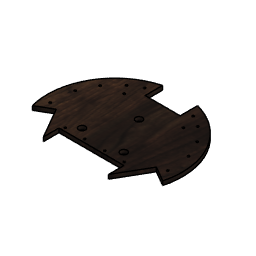
full_model (Autodesk Fusion 360 archive; units mm, degrees)
design "top"
Autodesk Fusion 360 part; units mm, degrees
sketch "Sketch1" plane through (0, 0, 0) normal (0, 0, 1) x (1, 0, 0)
  circle A0 centre (36, 80) radius 1.5
  line L0 (70.6242, -70.7971) -> (48.2374, -57.8721)
  circle A1 centre (87.282, -8.8231) radius 1.5
  circle A2 centre (51.282, -71.1769) radius 1.5
  circle A3 centre (-52.8772, 70) radius 1.5
  line L1 (0, 140) -> (0, -110) construction
  circle A4 centre (-36, 80) radius 1.5
  circle A5 centre (72.0833, 50) radius 1.5
  line L2 (-26, 96.5609) -> (26, 96.5609)
  circle A6 centre (52.8772, 70) radius 1.5
  line L3 (150, 0) -> (-170, 0) construction
  line L4 (-48.2374, -57.8721) -> (-70.6242, -70.7971)
  line L5 (26, 96.5609) -> (26, 70.7109)
  circle A7 centre (-51.282, -71.1769) radius 1.5
  circle A8 centre (-87.282, -8.8231) radius 1.5
  line L6 (-96.6242, -25.7638) -> (-74.2374, -12.8388)
  line L7 (48.2374, -57.8721) -> (74.2374, -12.8388)
  circle A9 centre (0, 0) radius 87.7268 construction
  line L8 (96.6242, -25.7638) -> (70.6242, -70.7971)
  line L9 (-74.2374, -12.8388) -> (-48.2374, -57.8721)
  line L10 (74.2374, -12.8388) -> (96.6242, -25.7638)
  circle A10 centre (84.0892, 25) radius 1.5
  circle A11 centre (0, 0) radius 100
  line L11 (-70.6242, -70.7971) -> (-96.6242, -25.7638)
  line L12 (26, 70.7109) -> (-26, 70.7109)
  circle A12 centre (-84.0892, 25) radius 1.5
  circle A13 centre (-72.0833, 50) radius 1.5
  line L13 (-26, 70.7109) -> (-26, 96.5609)
  line L14 (-48.2374, -57.8721) -> (48.2374, -57.8721)
  line L15 (48.2374, -57.8721) -> (48.2374, -87.5965)
  line L16 (48.2374, -87.5965) -> (-48.2374, -87.5965)
  line L17 (-48.2374, -87.5965) -> (-48.2374, -57.8721)
  circle A14 centre (0, 35.7109) radius 5
  circle A15 centre (-30.9265, -17.8554) radius 5
  circle A16 centre (30.9265, -17.8554) radius 5
  circle A17 centre (-15, -30) radius 1.5
  circle A18 centre (15, -30) radius 1.5
  circle A19 centre (-15, -62.8721) radius 2
  circle A20 centre (-15, -42.8721) radius 2
  circle A21 centre (-43.84, -30) radius 1.5
  circle A22 centre (-43.84, 57.68) radius 1.5
  circle A23 centre (43.84, 57.68) radius 1.5
  circle A24 centre (43.84, -30) radius 1.5
  line L18 (-48.2374, -57.8721) -> (48.2374, -57.8721)
  line L19 (48.2374, -57.8721) -> (48.2374, -34.8721)
  line L20 (48.2374, -34.8721) -> (-48.2374, -34.8721)
  line L21 (-48.2374, -34.8721) -> (-48.2374, -57.8721)
  dimension "d4" = 360
  dimension "d5" = 200
  dimension "d7" = 52
  dimension "d8" = 25.85
  dimension "d9" = 26
  dimension "d23" = 3
  dimension "d24" = 10
  dimension "d25" = 80
  dimension "d26" = 3
  dimension "d27" = 3
  dimension "d28" = 3
  dimension "d29" = 50
  dimension "d30" = 25
  dimension "d31" = 70
  dimension "d37" = 10
  dimension "d38" = 35
  dimension "d40" = 360
  dimension "d41" = 3
  dimension "d42" = 15
  dimension "d45" = 30
  dimension "d46" = 4
  dimension "d47" = 15
  dimension "d48" = 5
  dimension "d49" = 4
  dimension "d50" = 20
  dimension "d51" = 3
  dimension "d52" = 30
  dimension "d53" = 43.84
  dimension "d54" = 3
  dimension "d55" = 43.84
  dimension "d56" = 87.68
  dimension "d57" = 23
  constraint coincident A9.centre A11.centre
  constraint vertical L1
  constraint horizontal L3
  constraint horizontal L2
  constraint vertical L5
  constraint horizontal L12
  constraint vertical L13
  constraint coincident L2.start A11
  constraint symmetric A0 L1 A4
  constraint concentric A9 A11
  constraint coincident A8.centre A9
  constraint coincident A12.centre A9
  constraint coincident A3.centre A9
  constraint coincident A13.centre A9
  constraint symmetric L1 A10 A12
  constraint symmetric A3 L1 A6
  constraint symmetric L1 A5 A13
  constraint perpendicular L14 L15
  constraint parallel L14 L16
  constraint parallel L15 L17
  constraint horizontal L14
  constraint coincident L1 A14.centre
  constraint symmetric L1 A17 A18
  constraint symmetric L1 A21 A24
  constraint symmetric L1 A22 A23
  constraint perpendicular L18 L19
  constraint parallel L18 L20
  constraint parallel L19 L21
  measures "d5" diameter of A11
  measures "d7" distance of L2.end L2.start
  measures "d8" distance of L2.start L12.end
  measures "d9" distance of L1 L13
  measures "d23" diameter of A4
  measures "d24" distance of A4.centre L13
  measures "d25" distance of A4.centre L3
  measures "d26" diameter of A12
  measures "d27" diameter of A3
  measures "d28" diameter of A13
  measures "d29" distance of A13.centre L3
  measures "d30" distance of A12.centre L3
  measures "d31" distance of A3.centre L3
  measures "d37" diameter of A14
  measures "d38" distance of L12 A14.centre
  measures "d41" diameter of A17
  measures "d42" distance of L1 A17.centre
  measures "d45" distance of L3 A17.centre
  measures "d46" diameter of A19
  measures "d47" distance of L1 A19.centre
  measures "d48" distance of L14 A19.centre
  measures "d49" diameter of A20
  measures "d50" distance of A19.centre A20.centre
  measures "d51" diameter of A21
  measures "d52" distance of L3 A21.centre
  measures "d53" distance of L1 A21.centre
  measures "d54" diameter of A22
  measures "d55" distance of L1 A22.centre
  measures "d56" distance of A21.centre A22.centre
  measures "d57" distance of L4.start L20.end
extrude "Extrude1" add sketch "Sketch1" along normal blind 6 contours L5 L6 L7 L9 L10 A11 L12 L13 L19 L20 L21
sketch "Sketch2" plane through (0, 0, 6) normal (0, 0, 1) x (-1, 0, 0)
  circle A0 centre (84.0892, -25) radius 1.5
  circle A1 centre (43.84, -57.68) radius 1.5
  circle A2 centre (-43.84, 30) radius 1.5
  circle A3 centre (-30.9265, 17.8554) radius 5
  circle A4 centre (0, -35.7109) radius 5
  circle A5 centre (43.84, 30) radius 1.5
  circle A6 centre (-15, 30) radius 1.5
  circle A7 centre (15, 30) radius 1.5
  circle A8 centre (-43.84, -57.68) radius 1.5
  circle A9 centre (30.9265, 17.8554) radius 5
  circle A10 centre (72.0833, -50) radius 1.5
  circle A11 centre (52.8772, -70) radius 1.5
  circle A12 centre (-84.0892, -25) radius 1.5
  circle A13 centre (87.282, 8.8231) radius 1.5
  circle A14 centre (-52.8772, -70) radius 1.5
  circle A15 centre (36, -80) radius 1.5
  circle A16 centre (-87.282, 8.8231) radius 1.5
  circle A17 centre (-36, -80) radius 1.5
  circle A18 centre (-72.0833, -50) radius 1.5
  line L0 (-48.2374, 57.8721) -> (-74.2374, 12.8388)
  line L1 (-74.2374, 12.8388) -> (-96.6242, 25.7638)
  arc A19 (-96.6242, 25.7638) -> (-26, -96.5609) centre (0, 0) ccw
  line L2 (-26, -96.5609) -> (-26, -70.7109)
  line L3 (-26, -70.7109) -> (26, -70.7109)
  line L4 (26, -70.7109) -> (26, -96.5609)
  arc A20 (26, -96.5609) -> (96.6242, 25.7638) centre (0, 0) ccw
  line L5 (96.6242, 25.7638) -> (74.2374, 12.8388)
  line L6 (74.2374, 12.8388) -> (48.2374, 57.8721)
  line L7 (48.2374, 57.8721) -> (48.2374, 34.8721)
  line L8 (48.2374, 34.8721) -> (-48.2374, 34.8721)
  line L9 (-48.2374, 34.8721) -> (-48.2374, 57.8721)
equation "d53 = ( 87.68 / 2 ) * 1 mm"

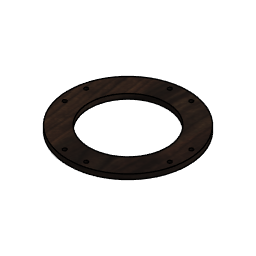
design "mirror_holder"
Autodesk Fusion 360 part; units mm, degrees
sketch "Sketch1" plane through (0, 0, 0) normal (0, 0, 1) x (1, 0, 0)
  circle A0 centre (0, 0) radius 50
  line L0 (0, 80) -> (0, -80) construction
  line L1 (-80, 0) -> (80, 0) construction
  circle A1 centre (-9, 44) radius 1.5
  circle A2 centre (-9, -44) radius 1.5
  circle A3 centre (-44, -9) radius 1.5
  circle A4 centre (44, -9) radius 1.5
  circle A5 centre (9, -44) radius 1.5
  circle A6 centre (9, 44) radius 1.5
  circle A7 centre (44, 9) radius 1.5
  circle A8 centre (-44, 9) radius 1.5
  circle A9 centre (0, 0) radius 32.5
  dimension "d1" = 100
  dimension "d2" = 3
  dimension "d3" = 9
  dimension "d4" = 44
  dimension "d5" = 3
  dimension "d6" = 9
  dimension "d7" = 44
  dimension "d9" = 360
  dimension "d12" = 65
  constraint coincident A0.centre A9.centre
  constraint vertical L0
  constraint horizontal L1
  constraint concentric A0 A9
  measures "d1" diameter of A0
  measures "d2" diameter of A1
  measures "d3" distance of L0 A1.centre
  measures "d4" distance of L1 A1.centre
  measures "d5" diameter of A2
  measures "d6" distance of L0 A2.centre
  measures "d7" distance of L1 A2.centre
  measures "d12" diameter of A9
extrude "Extrude1" add sketch "Sketch1" along normal blind 4
equation "d3 = ( ( 15 + 3 ) / 2 ) * 1 mm"
equation "d4 = ( 88 / 2 ) * 1 mm"

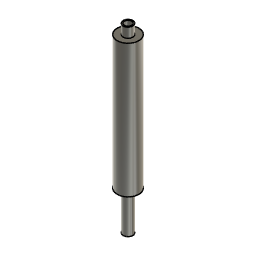
design "val"
Autodesk Fusion 360 part; units mm, degrees
sketch "Sketch1" plane through (0, 0, 0) normal (0, 0, 1) x (1, 0, 0)
  circle A0 centre (0, 0) radius 2
  circle A1 centre (0, 0) radius 4.5
  dimension "d1" = 4
  dimension "d2" = 9
  constraint coincident A0.centre A1.centre
  measures "d1" diameter of A0
  measures "d2" diameter of A1
extrude "Extrude1" add sketch "Sketch1" along normal blind 65 contours A0 | A1
extrude "Extrude2" cut sketch "Sketch1" along normal blind 10
extrude "Extrude3" add sketch "Sketch1" along normal blind 75 contours A0
sketch "Sketch2" plane through (0, 0, 75) normal (0, 0, 1) x (-1, 0, 0)
  circle A0 centre (0, 0) radius 2
  circle A1 centre (0, 0) radius 1.5
  dimension "d9" = 3
  constraint coincident A0.centre A1.centre
  measures "d9" diameter of A1
extrude "Extrude4" cut sketch "Sketch2" against normal blind 9 contours A1
extrude "Extrude5" cut 1 faces at (1.8203, -0.1739, 75) along direction (0, 0, -1) blind 6
extrude "Extrude6" add 1 faces at (0.637, 0.1965, 0) along direction (0, 0, -1) blind 6

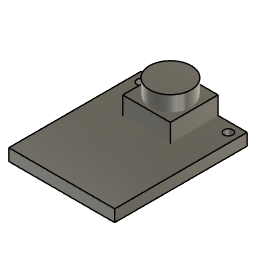
design "camera"
Autodesk Fusion 360 part; units mm, degrees
sketch "Sketch1" plane through (0, 0, 0) normal (0, 0, 1) x (1, 0, 0)
  line L0 (-17.78, 22.25) -> (17.78, 22.25)
  line L1 (17.78, 22.25) -> (17.78, -22.25)
  line L2 (17.78, -22.25) -> (-17.78, -22.25)
  line L3 (-17.78, -22.25) -> (-17.78, 22.25)
  line L4 (-17.78, 22.25) -> (17.78, -22.25) construction
  line L5 (17.78, 22.25) -> (-17.78, -22.25) construction
  circle A0 centre (-14.632, 19.102) radius 1.5
  line L6 (0, 50) -> (0, -35) construction
  circle A1 centre (14.632, 19.102) radius 1.5
  line L7 (8, 22.25) -> (-8, 22.25)
  line L8 (-8, 22.25) -> (-8, 6.25)
  line L9 (-8, 6.25) -> (8, 6.25)
  line L10 (8, 6.25) -> (8, 22.25)
  line L11 (8, 22.25) -> (-8, 6.25) construction
  line L12 (-8, 22.25) -> (8, 6.25) construction
  circle A2 centre (0, 14.25) radius 7
  point P0 (0, 14.25)
  dimension "d1" = 35.56
  dimension "d2" = 44.5
  dimension "d3" = 3
  dimension "d4" = 3.148
  dimension "d5" = 3.148
  dimension "d8" = 16
  dimension "d9" = 16
  dimension "d10" = 6.25
  dimension "d11" = 14
  constraint horizontal L0
  constraint perpendicular L0 L1
  constraint parallel L0 L2
  constraint parallel L1 L3
  constraint coincident L4 origin
  constraint coincident L5 origin
  constraint perpendicular L2 L6
  constraint symmetric A0 L6 A1
  constraint horizontal L7
  constraint perpendicular L7 L8
  constraint parallel L7 L9
  constraint parallel L8 L10
  constraint coincident L11 P0
  constraint coincident L12 P0
  constraint coincident L6 P0
  constraint coincident P0 A2.centre
  measures "d1" distance of L1.end L2.end
  measures "d2" distance of L0.end L1.end
  measures "d3" diameter of A0
  measures "d4" distance of L3 A0.centre
  measures "d5" distance of L0 A0.centre
  measures "d8" distance of L8.end L9.end
  measures "d9" distance of L7.end L8.end
  measures "d10" distance of origin L9
  measures "d11" diameter of A2
extrude "Extrude1" add sketch "Sketch1" along normal blind 4 contours L0 L1 L2 L3 L8 L9 L10 | L0 L7 L8 L9 L10 | A2 makes body 1
extrude "Extrude2" add sketch "Sketch1" along normal blind 10 separate body contours L0 L7 L8 L9 L10 | A2 makes body 2
extrude "Extrude3" add sketch "Sketch1" along normal blind 15 separate body contours A2 makes body 3
equation "d4 = 1.648 mm + ( 3 / 2 ) * 1 mm"
equation "d5 = 1.648 mm + ( 3 / 2 ) * 1 mm"
equation "d10 = ( 44.5 / 2 ) * 1 mm - 16 mm"

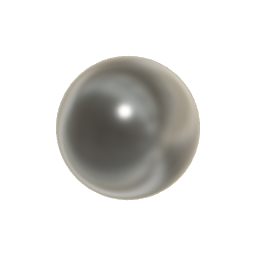
design "ball"
Autodesk Fusion 360 part; units mm, degrees
sphere "SpherePrimitive1" add diameter 74 placed x (0, 1, 0) y (0, 0, 1) z (1, 0, 0) at (0, 0, 0)

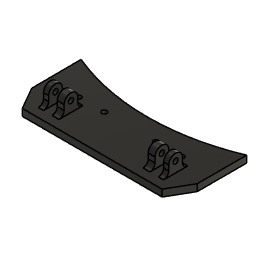
design "dribler_holder"
Autodesk Fusion 360 part; units mm, degrees
sketch "Sketch1" plane through (0, 0, 0) normal (0, 0, 1) x (1, 0, 0)
  line L0 (48.2374, 7.8721) -> (70.6242, 20.7971)
  line L1 (33.2374, -25.1279) -> (48.2374, 0.8529)
  circle A0 centre (-51.282, 21.1769) radius 1.5
  circle A1 centre (51.282, 21.1769) radius 1.5
  arc A2 (-55.6617, 33.0769) -> (-70.6242, 20.7971) centre (0, -50) ccw
  circle A3 centre (15, -20) radius 1.5
  line L2 (-33.2743, -25.1279) -> (33.2374, -25.1279)
  line L3 (-48.2374, 7.8721) -> (-48.2005, 0.8529)
  arc A4 (70.6242, 20.7971) -> (55.6617, 33.0769) centre (0, -50) ccw
  line L4 (-70.6242, 20.7971) -> (-48.2374, 7.8721)
  line L5 (-48.2005, 0.8529) -> (-33.2743, -25.1279)
  circle A5 centre (-15, -20) radius 1.5
  line L6 (48.2374, 0.8529) -> (48.2374, 7.8721)
  arc A6 (-55.6617, 33.0769) -> (55.6617, 33.0769) centre (0, 145) ccw
  line L7 (-40.7374, -12.1375) -> (40.7374, -12.1375)
  line L8 (48.2374, 7.8721) -> (48.2374, 29.6824)
  line L9 (-48.2374, 7.8721) -> (-48.3522, 29.7305)
  line L10 (0, -50) -> (0, 145) construction
  circle A7 centre (15, 10) radius 1.5
  circle A8 centre (30, 10) radius 1.5
  line L11 (126, 0) -> (-89, 0) construction
  line L12 (25, 5) -> (20, 5)
  line L13 (20, 5) -> (20, 15)
  line L14 (20, 15) -> (25, 15)
  line L15 (25, 15) -> (25, 5)
  line L16 (-25, 5) -> (-20, 5)
  line L17 (-20, 15) -> (-25, 15)
  line L18 (-25, 15) -> (-25, 5)
  line L19 (-20, 5) -> (-20, 15)
  circle A9 centre (-30, 10) radius 1.5
  circle A10 centre (-15, 10) radius 1.5
  line L20 (48.2374, 19.9303) -> (-48.3007, 19.9303)
  dimension "d57" = 3
  dimension "d58" = 3
  dimension "d59" = 10
  dimension "d60" = 10
  dimension "d61" = 5
  dimension "d62" = 20
  dimension "d63" = 5
  dimension "d64" = 5
  constraint midpoint L5 L7.start
  constraint midpoint L1 L7.end
  constraint parallel L2 L7
  constraint coincident A6 L8.end
  constraint perpendicular L7 L8
  constraint coincident A6 L9.end
  constraint parallel L3 L9
  constraint coincident A2.centre A4.centre
  constraint coincident A6.centre L10.end
  constraint vertical L10
  constraint horizontal L11
  constraint horizontal L12
  constraint vertical L13
  constraint horizontal L14
  constraint vertical L15
  constraint symmetric L10 A7 A10
  constraint symmetric L10 A8 A9
  constraint symmetric L10 L12.start L16.start
  constraint symmetric L10 L12.end L16.end
  constraint symmetric L10 L13.end L17.start
  constraint symmetric L10 L14.end L17.end
  constraint coincident L8 L20.start
  constraint coincident L9 L20.end
  constraint perpendicular L8 L20
  measures "d57" diameter of A7
  measures "d58" diameter of A8
  measures "d59" distance of A8.centre L11
  measures "d60" distance of A7.centre L11
  measures "d61" distance of L11 L12
  measures "d62" distance of L10 L13
  measures "d63" distance of A8.centre L15
  measures "d64" distance of A7.centre L13
extrude "Extrude7" add sketch "Sketch1" along normal blind 4 contours L1 L3 L5 L6 L7 L8 L9 L20 | A6 L8 L9 L20 | L12 L13 L14 L15 | L16 L17 L18 L19
extrude "Extrude8" add sketch "Sketch1" against normal blind 6 contours L12 L13 L14 L15 | L16 L17 L18 L19
sketch "Sketch5" plane through (0, 0, 4) normal (0, 0, 1) x (-1, 0, 0)
  circle A0 centre (30, -10) radius 1.5
  circle A1 centre (15, -10) radius 1.5
  circle A2 centre (-30, -10) radius 1.5
  circle A3 centre (-15, -10) radius 1.5
  line L0 (48.2005, -0.8529) -> (40.7374, 12.1375)
  line L1 (40.7374, 12.1375) -> (-40.7374, 12.1375)
  line L2 (-40.7374, 12.1375) -> (-48.2374, -0.8529)
  line L3 (-48.2374, -0.8529) -> (-48.2374, -29.6824)
  arc A4 (48.3522, -29.7305) -> (-48.2374, -29.6824) centre (0, -145) ccw
  line L4 (48.3522, -29.7305) -> (48.2005, -0.8529)
  line L5 (0, 35) -> (0, -35) construction
  line L6 (-36.5, 4) -> (-24.5, 4)
  line L7 (-24.5, 4) -> (-24.5, -4)
  line L8 (-24.5, -4) -> (-36.5, -4)
  line L9 (-36.5, -4) -> (-36.5, 4)
  line L10 (-36.5, 4) -> (-32.5, 4)
  line L11 (-32.5, 4) -> (-32.5, -4)
  line L12 (-32.5, -4) -> (-36.5, -4)
  line L13 (-36.5, -4) -> (-36.5, 4)
  line L14 (-24.5, 4) -> (-28.5, 4)
  line L15 (-28.5, 4) -> (-28.5, -4)
  line L16 (-28.5, -4) -> (-24.5, -4)
  line L17 (-24.5, -4) -> (-24.5, 4)
  line L18 (-100, 0) -> (80, 0) construction
  line L19 (24.5, 4) -> (24.5, -4)
  line L20 (28.5, -4) -> (24.5, -4)
  line L21 (24.5, -4) -> (36.5, -4)
  line L22 (36.5, 4) -> (32.5, 4)
  line L23 (36.5, -4) -> (36.5, 4)
  line L24 (36.5, -4) -> (36.5, 4)
  line L25 (32.5, -4) -> (36.5, -4)
  line L26 (32.5, 4) -> (32.5, -4)
  line L27 (28.5, 4) -> (28.5, -4)
  line L28 (24.5, 4) -> (28.5, 4)
  line L29 (36.5, 4) -> (24.5, 4)
  line L30 (24.5, -4) -> (24.5, 4)
  dimension "d69" = 12
  dimension "d70" = 8
  dimension "d71" = 4
  dimension "d72" = 8
  dimension "d73" = 4
  dimension "d74" = 8
  dimension "d75" = 32.5
  dimension "d76" = 4
  constraint vertical L5
  constraint horizontal L6
  constraint vertical L7
  constraint horizontal L8
  constraint vertical L9
  constraint horizontal L10
  constraint vertical L11
  constraint horizontal L12
  constraint vertical L13
  constraint horizontal L14
  constraint vertical L15
  constraint horizontal L16
  constraint vertical L17
  constraint perpendicular L13 L18
  constraint symmetric L5 L6.start L22.start
  constraint symmetric L5 L6.end L19.start
  constraint symmetric L5 L7.end L19.end
  constraint symmetric L5 L8.end L21.end
  constraint symmetric L5 L10.end L22.end
  constraint symmetric L5 L11.end L25.start
  constraint symmetric L5 L14.end L27.start
  constraint symmetric L5 L15.end L20.start
  measures "d69" distance of L6.start L6.end
  measures "d70" distance of L6.start L8.end
  measures "d71" distance of L6.start L10.end
  measures "d72" distance of L6.start L8.end
  measures "d73" distance of L6.end L14.end
  measures "d74" distance of L6.end L7.end
  measures "d75" distance of L5 L11
  measures "d76" distance of L6 L18
extrude "Extrude9" add sketch "Sketch5" along normal blind 10 contours L6 L8 L9 L10 L11 L12 L13 | L6 L7 L8 L14 L15 L16 L17 | L19 L20 L21 L27 L28 L29 L30 | L21 L22 L23 L24 L25 L26 L29
sketch "Sketch6" plane through (36.5, 0, 0) normal (1, 0, 0) x (0, 1, 0)
  line L0 (-4, 4) -> (4, 4)
  line L1 (4, 4) -> (4, 14)
  line L2 (4, 14) -> (-4, 14)
  line L3 (-4, 14) -> (-4, 4)
  line L4 (-4, 14) -> (4, 14)
  line L5 (4, 14) -> (4, 4)
  line L6 (4, 4) -> (-4, 4)
  line L7 (-4, 4) -> (-4, 14)
  circle A0 centre (0, 10) radius 1.5
  dimension "d79" = 3
  dimension "d80" = 4
  dimension "d81" = 4
  constraint horizontal L4
  constraint vertical L5
  constraint horizontal L6
  constraint vertical L7
  constraint coincident L0.end L1.start
  constraint coincident L2.end L3.start
  measures "d79" diameter of A0
  measures "d80" distance of L4 A0.centre
  measures "d81" distance of L5 A0.centre
extrude "Extrude10" cut sketch "Sketch6" against normal blind 170 contours A0
fillet "Fillet1" radius 4 8 edges at (34.5, -4, 14) (34.5, 4, 14) (26.5, -4, 14) (26.5, 4, 14) (-26.5, -4, 14) (-26.5, 4, 14) (-34.5, -4, 14) (-34.5, 4, 14)
fillet "Fillet2" radius 3 8 edges at (26.5, 4, 4) (34.5, 4, 4) (26.5, -4, 4) (34.5, -4, 4) (-34.5, -4, 4) (-26.5, -4, 4) (-34.5, 4, 4) (-26.5, 4, 4)
extrude "Extrude11" cut 1 faces at (-32.5, -0.0374, 6.6706) along direction (-1, 0, 0) blind 1
extrude "Extrude12" cut 1 faces at (32.5, 0.0374, 6.6706) along direction (1, 0, 0) blind 1
equation "d75 = ( 65 / 2 ) * 1 mm"
equation "d37 = 5 mm"
equation "d38 = d37"

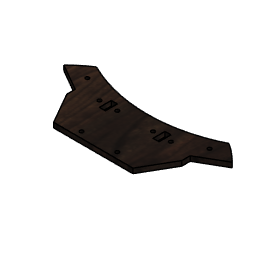
design "dribler"
Autodesk Fusion 360 part; units mm, degrees
sketch "Sketch1" plane through (0, 0, 0) normal (0, 0, 1) x (1, 0, 0)
  line L0 (-48.2374, 7.8721) -> (-48.2005, 0.8529)
  line L1 (20, 5) -> (20, 15)
  circle A0 centre (51.282, 21.1769) radius 1.5
  circle A1 centre (15, 10) radius 1.5
  circle A2 centre (-30, 10) radius 1.5
  line L2 (20, 15) -> (25, 15)
  line L3 (48.2374, 19.9303) -> (-48.3007, 19.9303)
  line L4 (25, 15) -> (25, 5)
  line L5 (-40.7374, -12.1375) -> (40.7374, -12.1375)
  line L6 (-25, 15) -> (-25, 5)
  line L7 (25, 5) -> (20, 5)
  line L8 (48.2374, 0.8529) -> (48.2374, 7.8721)
  line L9 (-20, 5) -> (-20, 15)
  line L10 (48.2374, 7.8721) -> (48.2374, 29.6824)
  arc A3 (-55.6617, 33.0769) -> (-70.6242, 20.7971) centre (0, -50) ccw
  circle A4 centre (-51.282, 21.1769) radius 1.5
  line L11 (48.2374, 7.8721) -> (70.6242, 20.7971)
  line L12 (-48.2005, 0.8529) -> (-33.2743, -25.1279)
  line L13 (33.2374, -25.1279) -> (48.2374, 0.8529)
  circle A5 centre (15, -20) radius 1.5
  arc A6 (-55.6617, 33.0769) -> (55.6617, 33.0769) centre (0, 145) ccw
  line L14 (-48.2374, 7.8721) -> (-48.3522, 29.7305)
  line L15 (-25, 5) -> (-20, 5)
  circle A7 centre (-15, 10) radius 1.5
  circle A8 centre (-15, -20) radius 1.5
  line L16 (-20, 15) -> (-25, 15)
  line L17 (-70.6242, 20.7971) -> (-48.2374, 7.8721)
  circle A9 centre (30, 10) radius 1.5
  line L18 (-33.2743, -25.1279) -> (33.2374, -25.1279)
  arc A10 (70.6242, 20.7971) -> (55.6617, 33.0769) centre (0, -50) ccw
  dimension "d63" = 3
  dimension "d64" = 3
  dimension "d65" = 5
  dimension "d66" = 5
  constraint midpoint L5.start L12
  constraint midpoint L5.end L13
  constraint parallel L5 L18
  constraint coincident L10.end A6
  constraint perpendicular L5 L10
  constraint coincident L14.end A6
  constraint parallel L0 L14
  constraint horizontal L7
  constraint vertical L1
  constraint horizontal L2
  constraint vertical L4
  constraint coincident L3.start L10
  constraint coincident L3.end L14
  constraint perpendicular L3 L10
  measures "d63" diameter of A1
  measures "d64" diameter of A9
  measures "d65" distance of A9.centre L4
  measures "d66" distance of A1.centre L1
extrude "Extrude3" add sketch "Sketch1" along normal blind 4
equation "d23 = 225 mm - 30 mm"

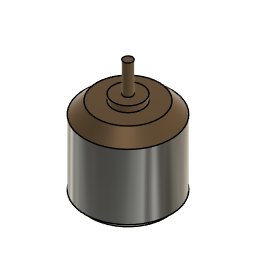
design "motor_1000KV"
Autodesk Fusion 360 part; units mm, degrees
sketch "Sketch1" plane through (0, 0, 0) normal (0, 0, 1) x (1, 0, 0)
  circle A0 centre (0, 0) radius 14.5
  line L0 (0, 30) -> (0, -25) construction
  line L1 (-30, 0) -> (26, 0) construction
  circle A1 centre (0, -10) radius 1.5
  circle A2 centre (10, 0) radius 1.5
  circle A3 centre (0, 10) radius 1.5
  circle A4 centre (-10, 0) radius 1.5
  dimension "d1" = 29
  dimension "d3" = 3
  dimension "d4" = 10
  dimension "d6" = 360
  constraint coincident A0.centre origin
  constraint vertical L0
  constraint horizontal L1
  constraint coincident L0 A1.centre
  measures "d1" diameter of A0
  measures "d3" diameter of A1
  measures "d4" distance of L1 A1.centre
extrude "Extrude1" add sketch "Sketch1" along normal blind 30
extrude "Extrude2" add sketch "Sketch1" along normal blind 30 contours A1 | A2 | A3 | A4
extrude "Extrude3" cut sketch "Sketch1" along normal blind 10 contours A1 | A2 | A3 | A4
sketch "Sketch2" plane through (0, 0, 30) normal (0, 0, 1) x (-1, 0, 0)
  circle A0 centre (0, 0) radius 14.5
  circle A1 centre (0, 0) radius 1.5
  dimension "d13" = 3
  constraint concentric A0 A1
  measures "d13" diameter of A1
extrude "Extrude4" add sketch "Sketch2" along normal blind 10 contours A1
extrude "Extrude5" cut 1 faces at (10.1127, -0.7204, 30) along direction (0, 0, -1) blind 2
sketch "Sketch3" plane through (0, 0, 28) normal (0, 0, 1) x (-1, 0, 0)
  circle A0 centre (0, 0) radius 1.5
  circle A1 centre (0, 0) radius 14.5
  circle A2 centre (0, 0) radius 5
  dimension "d18" = 10
  constraint coincident A0.centre A1.centre
  measures "d18" diameter of A2
extrude "Extrude6" add sketch "Sketch3" along normal blind 2 contours A2
chamfer "Chamfer1" distance 4 angle 45 1 edges at (-13.5187, 5.2434, 28)
chamfer "Chamfer2" distance 2 angle 45 1 edges at (-13.5187, -5.2434, 0)

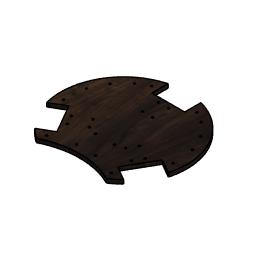
design "bottom"
Autodesk Fusion 360 part; units mm, degrees
sketch "Sketch1" plane through (0, 0, 0) normal (0, 0, 1) x (1, 0, 0)
  circle A0 centre (0, 0) radius 100
  line L0 (0, 140) -> (0, -110) construction
  line L1 (150, 0) -> (-170, 0) construction
  circle A1 centre (8, 63.1809) radius 1.5
  line L2 (-26, 96.5609) -> (26, 96.5609)
  line L3 (26, 96.5609) -> (26, 70.7109)
  line L4 (26, 70.7109) -> (-26, 70.7109)
  line L5 (-26, 70.7109) -> (-26, 96.5609)
  circle A2 centre (8, 37.7809) radius 1.5
  circle A3 centre (-8, 37.7809) radius 1.5
  circle A4 centre (-8, 63.1809) radius 1.5
  line L6 (-48.2374, -57.8721) -> (-70.6242, -70.7971)
  line L7 (-70.6242, -70.7971) -> (-96.6242, -25.7638)
  line L8 (-96.6242, -25.7638) -> (-74.2374, -12.8388)
  line L9 (-74.2374, -12.8388) -> (-48.2374, -57.8721)
  circle A5 centre (-58.7162, -24.6622) radius 1.5
  circle A6 centre (-36.7192, -11.9622) radius 1.5
  circle A7 centre (-28.7192, -25.8186) radius 1.5
  circle A8 centre (-50.7162, -38.5186) radius 1.5
  line L10 (74.2374, -12.8388) -> (96.6242, -25.7638)
  line L11 (96.6242, -25.7638) -> (70.6242, -70.7971)
  line L12 (70.6242, -70.7971) -> (48.2374, -57.8721)
  line L13 (48.2374, -57.8721) -> (74.2374, -12.8388)
  circle A9 centre (50.7162, -38.5186) radius 1.5
  circle A10 centre (28.7192, -25.8186) radius 1.5
  circle A11 centre (36.7192, -11.9622) radius 1.5
  circle A12 centre (58.7162, -24.6622) radius 1.5
  circle A13 centre (0, -195) radius 125
  circle A14 centre (-15, -60) radius 1.5
  circle A15 centre (-15, -30) radius 1.5
  circle A16 centre (15, -30) radius 1.5
  circle A17 centre (15, -60) radius 1.5
  circle A18 centre (-36, 80) radius 1.5
  circle A19 centre (36, 80) radius 1.5
  circle A20 centre (-87.282, -8.8231) radius 1.5
  circle A21 centre (-51.282, -71.1769) radius 1.5
  circle A22 centre (51.282, -71.1769) radius 1.5
  circle A23 centre (87.282, -8.8231) radius 1.5
  circle A24 centre (0, 0) radius 87.7268 construction
  circle A25 centre (-84.0892, 25) radius 1.5
  circle A26 centre (-52.8772, 70) radius 1.5
  circle A27 centre (-72.0833, 50) radius 1.5
  circle A28 centre (52.8772, 70) radius 1.5
  circle A29 centre (72.0833, 50) radius 1.5
  circle A30 centre (84.0892, 25) radius 1.5
  dimension "d1" = 200
  dimension "d2" = 3
  dimension "d3" = 52
  dimension "d4" = 25.85
  dimension "d6" = 26
  dimension "d7" = 7.53
  dimension "d8" = 8
  dimension "d9" = 3
  dimension "d10" = 25.4
  dimension "d11" = 8
  dimension "d13" = 360
  dimension "d15" = 250
  dimension "d16" = 195
  dimension "d17" = 3
  dimension "d18" = 15
  dimension "d19" = 60
  dimension "d20" = 3
  dimension "d21" = 15
  dimension "d22" = 30
  dimension "d25" = 3
  dimension "d26" = 10
  dimension "d27" = 80
  dimension "d29" = 360
  dimension "d30" = 3
  dimension "d31" = 3
  dimension "d32" = 3
  dimension "d33" = 50
  dimension "d34" = 25
  dimension "d35" = 70
  constraint coincident A0.centre A24.centre
  constraint vertical L0
  constraint horizontal L1
  constraint horizontal L2
  constraint vertical L3
  constraint horizontal L4
  constraint vertical L5
  constraint coincident A0 L2.start
  constraint symmetric L0 A1 A4
  constraint symmetric L0 A2 A3
  constraint symmetric L0 A14 A17
  constraint symmetric L0 A15 A16
  constraint symmetric L0 A18 A19
  constraint concentric A0 A24
  constraint coincident A20.centre A24
  constraint coincident A24 A25.centre
  constraint coincident A24 A26.centre
  constraint coincident A24 A27.centre
  constraint symmetric L0 A25 A30
  constraint symmetric L0 A26 A28
  constraint symmetric L0 A27 A29
  measures "d1" diameter of A0
  measures "d2" diameter of A1
  measures "d3" distance of L2.start L2.end
  measures "d4" distance of L2.start L4.end
  measures "d6" distance of L0 L5
  measures "d7" distance of A1.centre L4
  measures "d8" distance of L0 A1.centre
  measures "d9" diameter of A2
  measures "d10" distance of A1.centre A2.centre
  measures "d11" distance of L0 A2.centre
  measures "d15" diameter of A13
  measures "d16" distance of A0.centre A13.centre
  measures "d17" diameter of A14
  measures "d18" distance of L0 A14.centre
  measures "d19" distance of L1 A14.centre
  measures "d20" diameter of A15
  measures "d21" distance of L0 A15.centre
  measures "d22" distance of L1 A15.centre
  measures "d25" diameter of A18
  measures "d26" distance of L5 A18.centre
  measures "d27" distance of L1 A18.centre
  measures "d30" diameter of A25
  measures "d31" diameter of A26
  measures "d32" diameter of A27
  measures "d33" distance of L1 A27.centre
  measures "d34" distance of L1 A25.centre
  measures "d35" distance of L1 A26.centre
extrude "Extrude1" add sketch "Sketch1" along normal blind 6 contours A0 L3 L4 L5 L6 L8 L9 L10 L12 L13 A13
sketch "Sketch2" plane through (0, 0, 6) normal (0, 0, 1) x (-1, 0, 0)
  circle A0 centre (-36.7192, 11.9622) radius 1.5
  circle A1 centre (-15, 60) radius 1.5
  circle A2 centre (-50.7162, 38.5186) radius 1.5
  circle A3 centre (15, 30) radius 1.5
  circle A4 centre (50.7162, 38.5186) radius 1.5
  circle A5 centre (36.7192, 11.9622) radius 1.5
  circle A6 centre (-58.7162, 24.6622) radius 1.5
  circle A7 centre (15, 60) radius 1.5
  circle A8 centre (-28.7192, 25.8186) radius 1.5
  circle A9 centre (-15, 30) radius 1.5
  circle A10 centre (-72.0833, -50) radius 1.5
  circle A11 centre (-52.8772, -70) radius 1.5
  circle A12 centre (84.0892, -25) radius 1.5
  circle A13 centre (-36, -80) radius 1.5
  circle A14 centre (-51.282, 71.1769) radius 1.5
  circle A15 centre (72.0833, -50) radius 1.5
  circle A16 centre (87.282, 8.8231) radius 1.5
  circle A17 centre (36, -80) radius 1.5
  circle A18 centre (51.282, 71.1769) radius 1.5
  circle A19 centre (28.7192, 25.8186) radius 1.5
  circle A20 centre (-8, -63.1809) radius 1.5
  circle A21 centre (-84.0892, -25) radius 1.5
  circle A22 centre (-87.282, 8.8231) radius 1.5
  circle A23 centre (52.8772, -70) radius 1.5
  circle A24 centre (8, -37.7809) radius 1.5
  circle A25 centre (58.7162, 24.6622) radius 1.5
  circle A26 centre (-8, -37.7809) radius 1.5
  circle A27 centre (8, -63.1809) radius 1.5
  arc A28 (-55.6617, 83.0769) -> (-70.6242, 70.7971) centre (0, 0) ccw
  line L0 (-70.6242, 70.7971) -> (-48.2374, 57.8721)
  line L1 (-48.2374, 57.8721) -> (-74.2374, 12.8388)
  line L2 (-74.2374, 12.8388) -> (-96.6242, 25.7638)
  arc A29 (-96.6242, 25.7638) -> (-26, -96.5609) centre (0, 0) ccw
  line L3 (-26, -96.5609) -> (-26, -70.7109)
  line L4 (-26, -70.7109) -> (26, -70.7109)
  line L5 (26, -70.7109) -> (26, -96.5609)
  arc A30 (26, -96.5609) -> (96.6242, 25.7638) centre (0, 0) ccw
  line L6 (96.6242, 25.7638) -> (74.2374, 12.8388)
  line L7 (74.2374, 12.8388) -> (48.2374, 57.8721)
  line L8 (48.2374, 57.8721) -> (70.6242, 70.7971)
  arc A31 (70.6242, 70.7971) -> (55.6617, 83.0769) centre (0, 0) ccw
  arc A32 (-55.6617, 83.0769) -> (55.6617, 83.0769) centre (0, 195) ccw
equation "d6 = ( 52 / 2 ) * 1 mm"
equation "d8 = ( 16 / 2 ) * 1 mm"
equation "d16 = 225 mm - 30 mm"
equation "d33 = ( 200 / 2 / 2 ) * 1 mm"
equation "d34 = ( 200 / 2 / 2 / 2 ) * 1 mm"
equation "d35 = ( 200 / 2 / 2 / 2 ) * 1 mm + 45 mm"

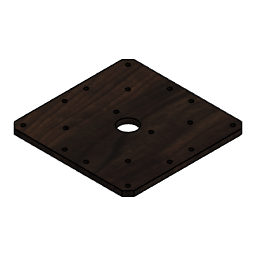
design "Combo_holder"
Autodesk Fusion 360 part; units mm, degrees
sketch "Sketch1" plane through (0, 0, 0) normal (0, 0, 1) x (1, 0, 0)
  line L0 (-8, 8) -> (8, -8) construction
  line L1 (50, -50) -> (50, 50)
  line L2 (-8, -8) -> (8, -8)
  line L3 (-8, 8) -> (-8, -8)
  line L4 (50, -45) -> (45, -50)
  line L5 (-50, 45) -> (-50, -50)
  circle A0 centre (-44, 9) radius 1.5
  circle A1 centre (9, -44) radius 1.5
  circle A2 centre (43.84, -43.84) radius 1.5
  circle A3 centre (-43.84, -43.84) radius 1.5
  line L6 (-50, -50) -> (50, -50)
  circle A4 centre (44, 9) radius 1.5
  circle A5 centre (-44, -9) radius 1.5
  circle A6 centre (43.84, 43.84) radius 1.5
  circle A7 centre (44, -9) radius 1.5
  line L7 (-90, 0) -> (90, 0) construction
  circle A8 centre (-43.84, 43.84) radius 1.5
  circle A9 centre (9, 44) radius 1.5
  line L8 (8, 8) -> (-8, -8) construction
  line L9 (-50, 50) -> (50, -50) construction
  circle A10 centre (0, 0) radius 7
  line L10 (50, 50) -> (-50, -50) construction
  circle A11 centre (-9, -44) radius 1.5
  line L11 (50, 50) -> (-45, 50)
  circle A12 centre (-9, 44) radius 1.5
  circle A13 centre (-14.632, 4.852) radius 1.5
  line L12 (8, 8) -> (-8, 8)
  circle A14 centre (14.632, 4.852) radius 1.5
  line L13 (-45, -50) -> (-50, -45)
  line L14 (-50, 45) -> (-45, 50)
  line L15 (8, -8) -> (8, 8)
  line L16 (45, 50) -> (50, 45)
  line L17 (-50, 50) -> (50, -50) construction
  circle A15 centre (-24.0138, -28.0138) radius 1.5
  line L18 (-50, 45) -> (-50, -50)
  line L19 (50, -45) -> (45, -50)
  line L20 (45, 50) -> (50, 45)
  line L21 (-90, 0) -> (90, 0) construction
  circle A16 centre (0, 0) radius 7.5
  circle A17 centre (43.84, -43.84) radius 1.5
  circle A18 centre (-25.9862, 25.9862) radius 1.5
  circle A19 centre (-43.84, -43.84) radius 1.5
  line L22 (-45, -50) -> (-50, -45)
  line L23 (50, 50) -> (-45, 50)
  line L24 (-50, 45) -> (-45, 50)
  line L25 (0, 80) -> (0, -100) construction
  line L26 (50, 50) -> (-50, -50) construction
  line L27 (50, -50) -> (50, 50)
  line L28 (-50, -50) -> (50, -50)
  circle A20 centre (43.84, 43.84) radius 1.5
  circle A21 centre (24.0138, 28.0138) radius 1.5
  circle A22 centre (25.9862, -25.9862) radius 1.5
  circle A23 centre (-43.84, 43.84) radius 1.5
  point P0 (0, 80)
  dimension "d2" = 360
  dimension "d4" = 360
  dimension "d6" = 360
  dimension "d7" = 100
  dimension "d8" = 100
  dimension "d9" = 5
  dimension "d10" = 5
  dimension "d11" = 3
  dimension "d12" = 43.84
  dimension "d13" = 3
  dimension "d14" = 16
  dimension "d15" = 16
  dimension "d16" = 14
  dimension "d17" = 3
  dimension "d18" = 3
  dimension "d20" = 360
  dimension "d22" = 360
  dimension "d23" = 100
  dimension "d24" = 100
  dimension "d25" = 5
  dimension "d26" = 5
  dimension "d27" = 3
  dimension "d28" = 43.84
  dimension "d29" = 43.84
  dimension "d30" = 15
  dimension "d31" = 3
  dimension "d32" = 3
  dimension "d33" = 73.5
  dimension "d34" = 3
  dimension "d35" = 54
  dimension "d36" = 50
  dimension "d37" = 36.75
  dimension "d38" = 3
  dimension "d39" = 54
  dimension "d40" = 50
  constraint horizontal L11
  constraint perpendicular L5 L11
  constraint parallel L6 L11
  constraint parallel L1 L5
  constraint coincident A10.centre L10
  constraint coincident A10.centre L9
  constraint coincident A10.centre A16.centre
  constraint coincident L9.start L5
  constraint coincident L9.start L11
  constraint horizontal L7
  constraint horizontal L12
  constraint perpendicular L3 L12
  constraint parallel L2 L12
  constraint parallel L3 L15
  constraint coincident A10.centre L8
  constraint coincident A10.centre L0
  constraint coincident A10.centre L7
  constraint horizontal L23
  constraint perpendicular L18 L23
  constraint parallel L23 L28
  constraint parallel L18 L27
  constraint coincident A10.centre L26
  constraint coincident A10.centre L17
  constraint coincident L9.start L18
  constraint coincident L9.start L23
  constraint horizontal L21
  constraint perpendicular L23 L25
  constraint coincident A18.centre L17
  constraint coincident A22.centre L17
  measures "d7" distance of L5.end L1.start
  measures "d8" distance of L9.start L5.end
  measures "d9" distance of L9.start L5.start
  measures "d10" distance of L9.start L11.end
  measures "d11" diameter of A3
  measures "d12" distance of A3.centre L7
  measures "d13" diameter of A13
  measures "d14" distance of L2.start L0.end
  measures "d15" distance of L0.start L2.start
  measures "d16" diameter of A10
  measures "d17" diameter of A12
  measures "d18" diameter of A11
  measures "d23" distance of L5.end L1.start
  measures "d24" distance of L5.end L9.start
  measures "d25" distance of L9.start L5.start
  measures "d26" distance of L11.end L9.start
  measures "d27" diameter of A19
  measures "d28" distance of A3.centre L21
  measures "d29" distance of A3.centre L25
  measures "d30" diameter of A16
  measures "d31" diameter of A18
  measures "d32" diameter of A22
  measures "d33" distance of A22.centre A18.centre
  measures "d34" diameter of A15
  measures "d35" vertical distance of A18.centre A15.centre
  measures "d36" horizontal distance of A22.centre A15.centre
  measures "d37" distance of A10.centre A18.centre
  measures "d38" diameter of A21
  measures "d39" vertical distance of A22.centre A21.centre
  measures "d40" horizontal distance of A18.centre A21.centre
extrude "Extrude1" add sketch "Sketch1" along normal blind 4 contours L1 L4 L5 L6 L11 L13 L14 L16 L18 L19 L20 L22 L23 L24 L27 L28 | L2 L3 L12 L15
sketch "Sketch2" plane through (0, 0, 4) normal (0, 0, 1) x (-1, 0, 0)
  circle A0 centre (-43.84, -43.84) radius 1.5
  circle A1 centre (43.84, 43.84) radius 1.5
  circle A2 centre (44, -9) radius 1.5
  circle A3 centre (9, 44) radius 1.5
  circle A4 centre (25.9862, -25.9862) radius 1.5
  circle A5 centre (-25.9862, 25.9862) radius 1.5
  circle A6 centre (9, -44) radius 1.5
  circle A7 centre (14.632, -4.852) radius 1.5
  circle A8 centre (-14.632, -4.852) radius 1.5
  circle A9 centre (43.84, -43.84) radius 1.5
  circle A10 centre (0, 0) radius 7.5
  circle A11 centre (24.0138, 28.0138) radius 1.5
  circle A12 centre (-24.0138, -28.0138) radius 1.5
  circle A13 centre (-43.84, 43.84) radius 1.5
  circle A14 centre (-9, -44) radius 1.5
  circle A15 centre (-44, -9) radius 1.5
  circle A16 centre (-9, 44) radius 1.5
  circle A17 centre (44, 9) radius 1.5
  circle A18 centre (-44, 9) radius 1.5
  line L0 (-50, 45) -> (-50, -45)
  line L1 (-50, -45) -> (-45, -50)
  line L2 (-45, -50) -> (45, -50)
  line L3 (45, -50) -> (50, -45)
  line L4 (50, -45) -> (50, 45)
  line L5 (50, 45) -> (45, 50)
  line L6 (45, 50) -> (-45, 50)
  line L7 (-45, 50) -> (-50, 45)

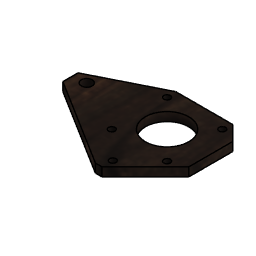
design "dribler_polovinka"
Autodesk Fusion 360 part; units mm, degrees
sketch "Sketch1" plane through (0, 0, 0) normal (0, 0, 1) x (1, 0, 0)
  line L0 (-119.7889, 0) -> (120, 0) construction
  line L1 (0, 100) -> (0, -100) construction
  circle A0 centre (0, 0) radius 10
  circle A1 centre (0, -25) radius 1.5
  circle A2 centre (-12.7279, 12.7279) radius 1.5
  circle A3 centre (-12.7279, -12.7279) radius 1.5
  circle A4 centre (12.7279, -12.7279) radius 1.5
  circle A5 centre (12.7279, 12.7279) radius 1.5
  circle A6 centre (-37, 0) radius 2.5
  line L2 (0, -30) -> (-3, -30)
  line L3 (-43, -5) -> (-43, 2)
  line L4 (-13, 17) -> (13.25, 17)
  line L5 (20, 10.25) -> (20, -10)
  line L6 (0, -30) -> (20, -10)
  line L7 (-3, -30) -> (-43, -5)
  line L8 (-43, 2) -> (-13, 17)
  line L9 (13.25, 17) -> (20, 10.25)
  point P0 (20, -30)
  point P1 (-43, -30)
  point P2 (-43, 17)
  point P3 (20, 17)
  dimension "d21" = 20
  dimension "d22" = 3
  dimension "d23" = 25
  dimension "d26" = 5
  dimension "d27" = 37
  dimension "d28" = 63
  dimension "d29" = 47
  dimension "d30" = 20
  dimension "d31" = 20
  dimension "d32" = 40
  dimension "d33" = 25
  dimension "d34" = 15
  dimension "d35" = 30
  dimension "d36" = 6.75
  dimension "d37" = 6.75
  constraint horizontal L0
  constraint vertical L1
  constraint coincident A0.centre origin
  constraint coincident L1 A1.centre
  constraint coincident L0 A6.centre
  constraint horizontal L2
  constraint vertical L3
  constraint horizontal L4
  constraint vertical L5
  constraint coincident P0 L2
  constraint coincident P0 L5
  constraint coincident P1 L2
  constraint coincident P1 L3
  constraint coincident P2 L3
  constraint coincident P2 L4
  constraint coincident P3 L4
  constraint coincident P3 L5
  measures "d21" diameter of A0
  measures "d22" diameter of A1
  measures "d23" distance of A0.centre A1.centre
  measures "d26" diameter of A6
  measures "d27" distance of A0.centre A6.centre
  measures "d28" distance of P0 P1
  measures "d29" distance of P0 P3
  measures "d30" distance of P0 L2.start
  measures "d31" distance of P0 L5.end
  measures "d32" distance of P1 L2.end
  measures "d33" distance of P1 L3.start
  measures "d34" distance of P2 L3.end
  measures "d35" distance of P2 L4.start
  measures "d36" distance of P3 L4.end
  measures "d37" distance of P3 L5.start
extrude "Extrude1" add sketch "Sketch1" along normal blind 4
equation "d31 = d30"
equation "d37 = d36"

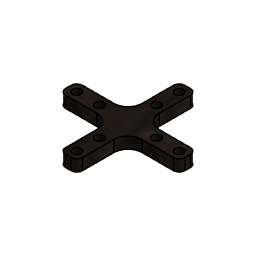
design "motor_holder"
Autodesk Fusion 360 part; units mm, degrees
sketch "Sketch1" plane through (0, 0, 0) normal (0, 0, 1) x (1, 0, 0)
  line L0 (0, 80) -> (0, -60) construction
  line L1 (-100, 0) -> (100, 0) construction
  circle A0 centre (0, 10) radius 1.5
  circle A1 centre (-10, 0) radius 1.5
  circle A2 centre (0, -10) radius 1.5
  circle A3 centre (10, 0) radius 1.5
  line L2 (1, 21) -> (-1, 21)
  line L3 (-3, 19) -> (-3, 8)
  line L4 (-1, -21) -> (1, -21)
  line L5 (3, 8) -> (3, 19)
  line L6 (3, 21) -> (-3, -21) construction
  line L7 (-3, 21) -> (3, -21) construction
  line L8 (-8, -3) -> (-19, -3)
  line L9 (-21, -1) -> (-21, 1)
  line L10 (-19, 3) -> (-8, 3)
  line L11 (21, 1) -> (21, -1)
  line L12 (21, -3) -> (-21, 3) construction
  line L13 (-21, -3) -> (21, 3) construction
  arc A4 (-1, 21) -> (-3, 19) centre (-1, 19) ccw
  arc A5 (3, 19) -> (1, 21) centre (1, 19) ccw
  arc A6 (1, -21) -> (3, -19) centre (1, -19) ccw
  arc A7 (-3, -19) -> (-1, -21) centre (-1, -19) ccw
  arc A8 (-21, -1) -> (-19, -3) centre (-19, -1) ccw
  arc A9 (-19, 3) -> (-21, 1) centre (-19, 1) ccw
  arc A10 (21, 1) -> (19, 3) centre (19, 1) ccw
  arc A11 (19, -3) -> (21, -1) centre (19, -1) ccw
  arc A12 (-8, 3) -> (-3, 8) centre (-8, 8) ccw
  line L14 (-3, -19) -> (-3, -8)
  line L15 (19, 3) -> (8, 3)
  arc A13 (3, 8) -> (8, 3) centre (8, 8) ccw
  line L16 (3, -19) -> (3, -8)
  arc A14 (-3, -8) -> (-8, -3) centre (-8, -8) ccw
  line L17 (8, -3) -> (19, -3)
  arc A15 (8, -3) -> (3, -8) centre (8, -8) ccw
  circle A16 centre (0, -18) radius 1.5
  circle A17 centre (18, 0) radius 1.5
  circle A18 centre (0, 18) radius 1.5
  circle A19 centre (-18, 0) radius 1.5
  dimension "d1" = 3
  dimension "d2" = 10
  dimension "d4" = 360
  dimension "d5" = 6
  dimension "d6" = 42
  dimension "d7" = 42
  dimension "d8" = 6
  dimension "d9" = 2
  dimension "d10" = 2
  dimension "d11" = 5
  dimension "d12" = 5
  dimension "d13" = 5
  dimension "d14" = 5
  dimension "d15" = 3
  dimension "d16" = 18
  dimension "d18" = 360
  constraint vertical L0
  constraint horizontal L1
  constraint coincident L0 A0.centre
  constraint horizontal L2
  constraint perpendicular L2 L3
  constraint parallel L2 L4
  constraint parallel L3 L5
  constraint coincident L6 origin
  constraint coincident L7 origin
  constraint horizontal L8
  constraint perpendicular L8 L9
  constraint parallel L8 L10
  constraint parallel L9 L11
  constraint coincident L12 origin
  constraint coincident L13 origin
  constraint coincident L7.start L2
  constraint coincident L7.start L3
  constraint tangent L2 A4
  constraint tangent L3 A4
  constraint coincident L6.start L2
  constraint coincident L6.start L5
  constraint tangent L2 A5
  constraint tangent L5 A5
  constraint equal A4 A5
  constraint coincident L7.end L5
  constraint coincident L7.end L4
  constraint tangent L5 A6
  constraint tangent L4 A6
  constraint equal A4 A6
  constraint coincident L6.end L3
  constraint coincident L6.end L4
  constraint tangent L3 A7
  constraint tangent L4 A7
  constraint equal A4 A7
  constraint coincident L13.start L8
  constraint coincident L13.start L9
  constraint tangent L8 A8
  constraint tangent L9 A8
  constraint equal A4 A8
  constraint coincident L12.end L10
  constraint coincident L12.end L9
  constraint tangent L10 A9
  constraint tangent L9 A9
  constraint equal A4 A9
  constraint coincident L13.end L10
  constraint coincident L13.end L11
  constraint tangent L10 A10
  constraint tangent L11 A10
  constraint equal A4 A10
  constraint coincident L12.start L8
  constraint coincident L12.start L11
  constraint tangent L8 A11
  constraint tangent L11 A11
  constraint coincident L10 A10.end
  constraint coincident L3 A7.start
  constraint tangent L10 A12
  constraint tangent L3 A12
  constraint tangent A7 L14
  constraint tangent A10 L15
  constraint coincident L5 A6.end
  constraint tangent L5 A13
  constraint tangent L15 A13
  constraint tangent A6 L16
  constraint coincident L8 A11.start
  constraint tangent L8 A14
  constraint tangent L14 A14
  constraint tangent L16 A15
  constraint tangent L17 A15
  constraint coincident L0 A16.centre
  measures "d1" diameter of A0
  measures "d2" distance of L1 A0.centre
  measures "d5" distance of L6.end L7.end
  measures "d6" distance of L7.start L6.end
  measures "d7" distance of L12.end L13.end
  measures "d8" distance of L13.start L12.end
  measures "d9" radius of A4
  measures "d10" radius of A11
  measures "d11" radius of A12
  measures "d12" radius of A13
  measures "d13" radius of A14
  measures "d14" radius of A15
  measures "d15" diameter of A16
  measures "d16" distance of origin A16.centre
extrude "Extrude1" add sketch "Sketch1" along normal blind 4
equation "d7 = ( ( 18 + 3 ) * 2 ) * 1 mm"
